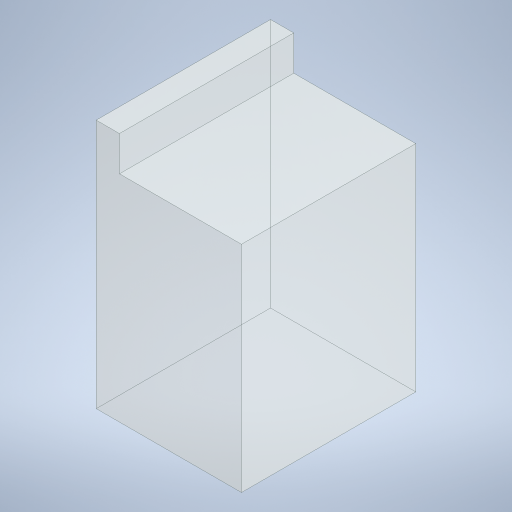
# Autodesk Inventor part: Stove
Saved by Autodesk Inventor 2024 (Build 280153000, 153)
## iProperties
Created: 2023-03-29
Part Number: Stove
Material: Steel
Document SubType Name: Modeling
Designer: Tom
Density: 7.85 g/cm^3
Appearance: Clear
Author: Tom
Autodesk Inventor part; units mm, degrees
ref_plane "YZ Plane" through (0, 0, 0) normal (1, 0, 0) x (0, 1, 0)
ref_plane "XZ Plane" through (0, 0, 0) normal (0, 1, 0) x (-1, 0, 0)
ref_plane "XY Plane" through (0, 0, 0) normal (0, 0, 1) x (1, 0, 0)
sketch "Sketch1" plane through (0, 0, 0) normal (0, 1, 0) x (-1, 0, 0)
  line L0 (0, 0) -> (-635, 0)
  line L1 (-635, 0) -> (-635, -762)
  line L2 (-635, -762) -> (0, -762)
  line L3 (0, -762) -> (0, 0)
  dimension "d4" = 762
  dimension "d5" = 635
  constraints: 8 end point, 2 parallel, 1 horizontal, 1 perpendicular
  measures "d4" distance of L2.end L0.start
  measures "d5" distance of L1.end L2.end
extrude "Extrusion1" add sketch "Sketch1" along normal blind 939.8
sketch "Sketch2" plane through (0, 939.8, 0) normal (0, 1, 0) x (1, 0, 0)
  line L0 (0, 762) -> (0, 0) projected
  line L1 (0, 0) -> (635, 0) projected
  line L2 (0, 762) -> (101.6, 762)
  line L3 (101.6, 762) -> (101.6, 0)
  line L4 (101.6, 0) -> (0, 0)
  line L5 (0, 0) -> (0, 762)
  dimension "d6" = 101.6
  constraints: 8 end point, 2 parallel, 1 horizontal, 1 perpendicular, 1 point on line
  measures "d6" distance between parallel lines of L0 L3
extrude "Extrusion2" add sketch "Sketch2" along normal blind 152.4
body "Solid1"
